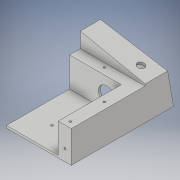
# Autodesk Inventor part: CPLRightOne
Saved by Autodesk Inventor 2019 (Build 230136000, 136)
## iProperties
Created: 2019-01-04
Part Number: CPLRightOne
Material: Generic
Document SubType Name: Modeling
Designer: james
Density: 1 g/cm^3
Appearance: Default
Author: james
Autodesk Inventor part; units mm, degrees
ref_plane "YZ Plane" through (0, 0, 0) normal (1, 0, 0) x (0, 1, 0)
ref_plane "XZ Plane" through (0, 0, 0) normal (0, 1, 0) x (-1, 0, 0)
ref_plane "XY Plane" through (0, 0, 0) normal (0, 0, 1) x (1, 0, 0)
sketch "Sketch1" plane through (0, 0, 0) normal (0, 1, 0) x (-1, 0, 0)
  line L0 (99.052281, 106.212918) -> (-21.597719, 106.212918)
  line L1 (-21.597719, 106.212918) -> (-21.597719, -39.837082)
  line L2 (-21.597719, -39.837082) -> (99.052281, -39.837082)
  line L3 (99.052281, -39.837082) -> (99.052281, 106.212918)
  point P0 (0, 0)
  dimension "d0" = 146.05
  dimension "d1" = 120.65
  constraints: 8 end point, 2 parallel, 1 horizontal, 1 perpendicular
  measures "d0" distance of L0.end L1.end
  measures "d1" distance of L1.end L2.end
extrude "Extrusion1" add sketch "Sketch1" along normal blind 5.08
sketch "Sketch2" plane through (21.597719, 0, 106.212918) normal (1, 0, 0) x (0, 0, -1)
  line L0 (0, 5.08) -> (146.05, 5.08) projected
  line L1 (146.05, 5.08) -> (140.97, 5.08)
  line L2 (140.97, 5.08) -> (140.97, 71.12)
  line L3 (140.97, 71.12) -> (146.05, 71.12)
  line L4 (146.05, 71.12) -> (146.05, 5.08)
  line L5 (0, 0) -> (146.05, 0) projected
  point P0 (106.212918, 0)
  dimension "d4" = 5.08
  dimension "d5" = 71.12
  constraints: 8 end point, 2 parallel, 1 horizontal, 1 perpendicular
  measures "d4" distance between parallel lines of L2 L4
  measures "d5" distance between parallel lines of L3 L5
extrude "Extrusion2" add sketch "Sketch2" against normal blind 120.65
sketch "Sketch3" plane through (-99.052281, 0, 106.212918) normal (0, 0, 1) x (1, 0, 0)
  line L0 (0, 5.08) -> (120.65, 5.08) projected
  line L1 (120.65, 5.08) -> (115.57, 5.08)
  line L2 (115.57, 5.08) -> (115.57, 71.12)
  line L3 (115.57, 71.12) -> (120.65, 71.12)
  line L4 (120.65, 71.12) -> (120.65, 5.08)
  line L5 (0, 0) -> (120.65, 0) projected
  point P0 (99.052281, 0)
  dimension "d8" = 5.08
  dimension "d9" = 71.12
  constraints: 8 end point, 2 parallel, 1 horizontal, 1 perpendicular
  measures "d8" distance between parallel lines of L4 L2
  measures "d9" distance between parallel lines of L3 L5
extrude "Extrusion3" add sketch "Sketch3" against normal blind 146.05
sketch "Sketch4" plane through (-99.052281, 0, 106.212918) normal (0, 0, 1) x (1, 0, 0)
  line L0 (115.57, 5.08) -> (115.57, 71.12) projected
  line L1 (115.57, 71.12) -> (120.65, 71.12) projected
  line L2 (115.57, 71.12) -> (139.7, 71.12)
  line L3 (139.7, 71.12) -> (139.7, 66.04)
  line L4 (139.7, 66.04) -> (115.57, 66.04)
  line L5 (115.57, 66.04) -> (115.57, 71.12)
  point P0 (99.052281, 0)
  dimension "d12" = 5.08
  dimension "d13" = 24.13
  constraints: 8 end point, 2 parallel, 1 horizontal, 1 perpendicular
  measures "d12" distance between parallel lines of L4 L2
  measures "d13" distance of L0.end L2.end
extrude "Extrusion4" add sketch "Sketch4" against normal blind 165.1
sketch "Sketch5" plane through (-99.052281, 0, -39.837082) normal (-1, 0, 0) x (0, 0, 1)
  line L0 (5.08, 5.08) -> (5.08, 71.12) projected
  line L1 (5.08, 71.12) -> (0, 71.12) projected
  line L2 (5.08, 71.12) -> (-19.05, 71.12)
  line L3 (-19.05, 71.12) -> (-19.05, 66.04)
  line L4 (-19.05, 66.04) -> (5.08, 66.04)
  line L5 (5.08, 66.04) -> (5.08, 71.12)
  point P0 (39.837082, 0)
  dimension "d16" = 5.08
  dimension "d17" = 24.13
  constraints: 8 end point, 2 parallel, 1 horizontal, 1 perpendicular
  measures "d16" distance between parallel lines of L4 L2
  measures "d17" distance of L0.end L2.end
extrude "Extrusion5" add sketch "Sketch5" against normal blind 139.7
sketch "Sketch7" plane through (-99.052281, 0, -58.887082) normal (0, 0, -1) x (-1, 0, 0)
  line L0 (-139.7, 71.12) -> (-144.78, 71.12)
  line L1 (-144.78, 71.12) -> (-144.78, 0)
  line L2 (-144.78, 0) -> (-139.7, 0)
  line L3 (-139.7, 0) -> (-139.7, 71.12)
  line L4 (-139.7, 71.12) -> (-139.7, 66.04) projected
  point P0 (-99.052281, 0)
  dimension "d26" = 5.08
  dimension "d27" = 0
  dimension "d28" = 71.12
  constraints: 8 end point, 2 parallel, 1 horizontal, 1 perpendicular
  measures "d26" distance between parallel lines of L1 L3
  measures "d27" distance between parallel lines of L4 L3
  measures "d28" distance between parallel lines of L0 L2
extrude "Extrusion7" add sketch "Sketch7" against normal blind 165.1
sketch "Sketch8" plane through (-99.052281, 0, -39.837082) normal (-1, 0, 0) x (0, 0, 1)
  line L0 (-77.47, 0) -> (-82.55, 0)
  line L1 (146.05, 0) -> (146.05, 5.08)
  line L2 (-77.47, 0) -> (-55.076473, 127)
  line L3 (-19.05, 0) -> (-19.05, 66.04)
  line L4 (-55.076473, 127) -> (-60.156473, 127)
  line L5 (-60.156473, 127) -> (-82.55, 0)
  point P0 (39.837082, 0)
  dimension "d31" = 5.08
  dimension "d32" = 228.6
  dimension "d33" = 10
  dimension "d34" = 5.08
  dimension "d35" = 127
  constraints: 8 end point, 2 horizontal
  measures "d31" distance of L0.start L0.end
  measures "d32" distance from line of L0.end L1
  measures "d33" angle of L2 L3
  measures "d34" distance of L2.end L4.end
  measures "d35" distance between parallel lines of L0 L4
extrude "Extrusion8" add sketch "Sketch8" against normal blind 144.78
sketch "Sketch9" plane through (-99.052281, 0, -39.837082) normal (-1, 0, 0) x (0, 0, 1)
  line L0 (-19.05, 0) -> (-19.05, 66.04) projected
  line L1 (-19.05, 66.04) -> (-24.13, 66.04)
  line L2 (-24.13, 66.04) -> (-24.13, 142.24)
  line L3 (-24.13, 142.24) -> (-19.05, 142.24)
  line L4 (-19.05, 142.24) -> (-19.05, 66.04)
  point P0 (39.837082, 0)
  dimension "d38" = 76.2
  dimension "d39" = 5.08
  constraints: 8 end point, 2 parallel, 1 horizontal, 1 perpendicular
  measures "d38" distance of L3.end L0.end
  measures "d39" distance between parallel lines of L2 L4
extrude "Extrusion9" add sketch "Sketch9" against normal blind 144.78
sketch "Sketch13" plane through (-99.052281, 71.12, -58.887082) normal (0, 0, 1) x (1, 0, 0)
  line L0 (0, 55.88) -> (0, -71.12)
  line L1 (0, -71.12) -> (120.65, -71.12)
  line L2 (0, 34.1884) -> (-78.886299, 34.1884)
  line L3 (0, 34.1884) -> (158.447464, 1.144718)
  line L4 (0, 34.1884) -> (0, 135.397645)
  line L5 (0, 135.397645) -> (157.416456, 135.397645)
  line L6 (157.416456, 135.397645) -> (158.447464, 1.144718)
  point P0 (99.052281, -71.12)
  dimension "d51" = 168.22
  constraints: 10 end point, 1 horizontal, 1 perpendicular, 1 point on line, 1 vertical
  measures "d51" angle of L2 L3
extrude "Extrusion13" cut sketch "Sketch13" against normal blind 114.6175
sketch "Sketch26" plane through (0, 5.08, 0) normal (0, 1, 0) x (1, 0, 0)
  line L0 (-99.052281, 34.757082) -> (-99.052281, -106.212918)
  line L1 (-99.052281, -106.212918) -> (16.517719, -106.212918)
  point P0 (0, 0)
  point P1 (-48.252281, -55.412918)
  dimension "d93" = 50.8
  dimension "d94" = 50.8
  measures "d93" distance from line of L0 point (-48.252, -55.413)
  measures "d94" distance from line of L1 point (-48.252, -55.413)
hole "Hole3" at (-48.252281, 5.08, 55.412918) direction (0, -1, 0) diameter 4.826 end through all
sketch "Sketch29" plane through (45.727719, 0, -58.887082) normal (1, 0, 0) x (0, 0, -1)
  line L0 (45.175195, 75.115022) -> (58.42, 0)
  line L1 (5.08, 73.952952) -> (45.175195, 73.952952)
  line L2 (5.08, 66.04) -> (5.08, 75.115022)
  line L3 (0, 66.04) -> (5.08, 66.04)
  line L4 (0, 66.04) -> (0, 0)
  line L5 (-19.05, 0) -> (58.42, 0)
  point P0 (-58.887082, 0)
  point P1 (36.026473, 127)
  point P2 (5.08, 142.24)
sketch "Sketch29 outline for Extrusion22" plane through (45.727719, 0, -58.887082) normal (1, 0, 0) x (0, 0, -1)
  line L0 (45.175195, 75.115022) -> (58.42, 0)
  line L1 (58.42, 0) -> (0, 0)
  line L2 (0, 0) -> (0, 66.04)
  line L3 (0, 66.04) -> (5.08, 66.04)
  line L4 (5.08, 66.04) -> (5.08, 75.115022)
  line L5 (5.08, 75.115022) -> (45.175195, 75.115022)
extrude "Extrusion22" add sketch "Sketch29 outline for Extrusion22" against normal blind 5.08
sketch "Sketch38" plane through (-99.052281, 105.3084, -98.73837) normal (0.2041544, 0.9789387, 0) x (0.9789387, -0.2041544, 0)
  line L0 (147.894856, -34.771288) -> (147.894856, 5.323907)
  line L1 (147.894856, 5.323907) -> (147.894856, -34.772919)
  line L2 (142.921848, -34.771288) -> (142.921848, 5.323907)
  line L3 (147.894856, -34.772919) -> (3.742348, -34.772919)
  line L4 (8.016815, -34.771288) -> (144.774553, -34.771288)
  line L5 (3.742348, -34.772919) -> (3.742348, -0.025087)
  line L6 (3.742348, -0.025087) -> (3.742348, 2.656747)
  line L7 (3.742348, 2.656747) -> (147.804186, 7.842673)
  line L8 (0, 5.08) -> (147.894856, 10.403907)
  line L9 (147.894856, 10.403907) -> (147.894856, 5.323907)
  line L10 (147.804186, 7.842673) -> (147.894856, 5.323907)
  point P0 (118.46528, -98.73837)
  constraints: 10 end point, 2 parallel, 2 vertical, 1 horizontal, 1 perpendicular, 4 other
extrude "Extrusion30" add sketch "Sketch38" against normal blind 5.08
sketch "Sketch40" plane through (-99.052281, 0, -39.837082) normal (-1, 0, 0) x (0, 0, 1)
  line L0 (0, 0) -> (0, 66.04)
  line L1 (-24.13, 66.04) -> (0, 66.04)
  line L2 (-24.13, 66.04) -> (-24.13, 105.3084)
  line L3 (-58.901288, 105.3084) -> (-77.47, 0)
  line L4 (-19.05, 105.3084) -> (-24.13, 105.3084)
  line L5 (-24.13, 104.544383) -> (-59.036005, 104.544383)
  line L6 (-24.13, 105.3084) -> (-59.036005, 104.544383)
  line L7 (146.05, 0) -> (0, 0)
  line L8 (-77.47, 0) -> (146.05, 0)
  line L9 (0, 0) -> (-77.47, 0)
  point P0 (39.837082, 0)
  constraints: 4 end point, 1 horizontal
extrude "Extrusion31" add sketch "Sketch40" against normal blind 5.08 contours L8 L3 L5 L2 L1 L0
sketch "Sketch41" plane through (-99.052281, 104.544383, -63.967082) normal (0, 0, -1) x (-1, 0, 0)
  line L0 (-3.66353, 0) -> (0, 0)
  line L1 (0, 0) -> (0, 0.764017)
  line L2 (0, 0.764017) -> (-3.66353, 0)
  point P0 (-99.052281, -104.544383)
  point P1 (-5.08, -5.484693)
extrude "Extrusion32" add sketch "Sketch41" along normal blind 36.83
sketch "Sketch43" plane through (-99.052281, 71.12, -58.887082) normal (0, 0, 1) x (1, 0, 0)
  line L0 (5.08, 33.128983) -> (3.66353, 33.424383)
  line L1 (5.08, 33.424383) -> (5.08, 33.128983)
  line L2 (3.66353, 33.424383) -> (5.08, 33.424383)
  point P0 (99.052281, -71.12)
extrude "Extrusion33" cut sketch "Sketch43" against normal blind 41.5925
sketch "Sketch44" plane through (40.647719, 0, 106.212918) normal (-1, 0, 0) x (0, 0, 1)
  line L0 (0, 66.04) -> (-170.18, 66.04)
  line L1 (-170.18, 66.04) -> (-142.520317, 66.04)
  line L2 (-142.520317, 66.04) -> (-142.520317, 48.69089)
  line L3 (-142.520317, 48.69089) -> (-170.18, 66.04)
  point P0 (-106.212918, 0)
  constraints: 6 end point, 1 point on line, 1 vertical
extrude "Extrusion34" add sketch "Sketch44" along normal blind 135.255
sketch "Sketch47" plane through (-99.052281, 0, 106.212918) normal (0, 0, 1) x (1, 0, 0)
  line L0 (139.7, 66.04) -> (120.65, 66.04)
  line L1 (139.741198, 66.04) -> (120.65, 66.04)
  line L2 (120.65, 66.04) -> (139.741198, 59.182182)
  line L3 (139.741198, 59.182182) -> (139.741198, 66.04)
  line L4 (139.7, 0) -> (139.7, 70.985145)
  point P0 (99.052281, 0)
  constraints: 6 end point, 1 collinear, 1 parallel
extrude "Extrusion35" add sketch "Sketch47" against normal blind 143.1925
sketch "Sketch19" plane through (-99.052281, 71.12, -34.757082) normal (0, 1, 0) x (1, 0, 0)
  line L0 (144.78, 24.13) -> (0, 24.13) projected
  line L1 (115.57, -140.97) -> (115.57, 0) projected
  point P0 (99.052281, -34.757082)
  point P1 (130.175, -52.07)
  point P2 (130.175, -128.27)
  dimension "d63" = 76.2
  dimension "d64" = 14.605
  dimension "d65" = 14.605
  dimension "d66" = 76.2
  measures "d63" distance of point (130.175, -128.27) point (130.175, -52.07)
  measures "d64" distance from line of L1 point (130.175, -128.27)
  measures "d65" distance from line of L1 point (130.175, -52.07)
  measures "d66" distance from line of point (130.175, -52.07) L0
hole "Hole1" at (31.122719, 71.12, 17.312918) at (31.122719, 71.12, 93.512918) direction (0, -1, 0) diameter 4.826 end through all
sketch "Sketch20" plane through (-99.052281, 71.12, -34.757082) normal (0, 1, 0) x (1, 0, 0)
  line L0 (115.57, 0) -> (0, 0) projected
  circle A0 centre (130.175, -52.07) radius 2.413 projected
  point P0 (99.052281, -34.757082)
  point P1 (63.5, 14.605)
  dimension "d74" = 14.605
  dimension "d75" = 66.675
  measures "d74" distance from line of point (63.5, 14.605) L0
  measures "d75" horizontal distance of A0.centre point (63.5, 14.605)
hole "Hole2" at (-35.552281, 71.12, -49.362082) direction (0, -1, 0) diameter 4.826 end through all
sketch "Sketch48" plane through (-99.052281, 0, 106.212918) normal (0, 0, 1) x (1, 0, 0)
  line L0 (5.08, 66.04) -> (139.7, 66.04)
  line L1 (120.65, 66.04) -> (139.7, 59.196981)
  line L2 (139.7, 59.196981) -> (139.7, 0)
  line L3 (120.65, 0) -> (120.65, 66.04)
  line L4 (139.7, 0) -> (120.65, 0)
  line L5 (0, 0) -> (144.78, 0)
  point P0 (99.052281, 0)
  constraints: 2 end point, 1 collinear
extrude "Extrusion36" add sketch "Sketch48" against normal blind 5.08
sketch "Sketch49" plane through (-99.052281, 5.08, -34.757082) normal (-1, 0, 0) x (0, 0, 1)
  line L0 (0, 0) -> (0, 66.04) projected
  line L1 (140.97, -5.08) -> (-87.63, -5.08) projected
  point P0 (34.757082, -5.08)
  point P1 (-50.8, 20.32)
  point P2 (-50.8, 45.72)
  dimension "d152" = 50.8
  dimension "d153" = 50.8
  dimension "d154" = 25.4
  dimension "d155" = 25.4
  measures "d152" distance from line of L0 point (-50.8, 45.72)
  measures "d153" distance from line of L0 point (-50.8, 20.32)
  measures "d154" distance from line of L1 point (-50.8, 20.32)
  measures "d155" distance of point (-50.8, 45.72) point (-50.8, 20.32)
hole "Hole6" at (-99.052281, 25.4, -85.557082) at (-99.052281, 50.8, -85.557082) direction (1, 0, 0) diameter 4.826 depth 25.4 tip angle 118
sketch "Sketch50" plane through (-99.052281, 0, 106.212918) normal (0, 0, 1) x (1, 0, 0)
  line L0 (0, 0) -> (144.78, 0) projected
  line L1 (115.57, 5.08) -> (115.57, 71.12) projected
  point P0 (99.052281, 0)
  point P1 (130.81, 25.4)
  dimension "d163" = 25.4
  dimension "d164" = 15.24
  measures "d163" distance from line of point (130.81, 25.4) L0
  measures "d164" distance from line of L1 point (130.81, 25.4)
hole "Hole7" at (31.757719, 25.4, 106.212918) direction (0, 0, -1) diameter 4.826 depth 25.4 tip angle 118
sketch "Sketch51" plane through (45.727719, 75.115022, -58.887082) normal (0.2041544, 0.9789387, 0) x (0.9789387, -0.2041544, 0)
  line L0 (-147.894856, 44.931288) -> (0, 50.255195)
  line L1 (0, 0) -> (-147.894856, 0)
  line L2 (0, 50.255195) -> (0, 0)
  point P0 (-29.429576, -58.887082)
  point P1 (-34.205528, 24.13)
  dimension "d172" = 24.87775
  dimension "d173" = 24.13
  dimension "d174" = 34.20553
  measures "d172" distance from line of L0 point (-34.206, 24.13)
  measures "d173" distance from line of L1 point (-34.206, 24.13)
  measures "d174" distance from line of L2 point (-34.206, 24.13)
hole "Hole8" at (12.242604, 82.098229, -83.017082) direction (-0.2041544, -0.9789387, 0) diameter 15.875 depth 25.4 tip angle 118.1875
sketch "Sketch52" plane through (-99.052281, 5.08, -34.757082) normal (0, 0, 1) x (1, 0, 0)
  circle A0 centre (83.137068, 28.704927) radius 19.05
  point P0 (99.052281, -5.08)
  dimension "d182" = 38.1
  constraints: 1 centre point
  measures "d182" diameter of A0
extrude "Extrusion37" cut sketch "Sketch52" against normal blind 25.4
equation "\"d0\" = CPDLengthHole"
equation "\"d1\" = CPDWidthHole"
equation "\"d2\" = WallWidth"
equation "\"d4\" = WallWidth"
equation "\"d5\" = CPDeckHeight"
equation "\"d6\" = CPDWidthHole"
equation "\"d8\" = WallWidth"
equation "\"d9\" = CPDeckHeight"
equation "\"d10\" = CPDLengthHole"
equation "\"d12\" = WallWidth"
equation "\"d13\" = WallWidth + ControlPlateShelfLength"
equation "\"d14\" = CPDLengthHole + ControlPlateShelfLength"
equation "\"d16\" = WallWidth"
equation "\"d17\" = WallWidth + ControlPlateShelfLength"
equation "\"d18\" = CPDWidthHole + ControlPlateShelfLength"
equation "\"d26\" = WallWidth"
equation "\"d28\" = CPDeckHeight"
equation "\"d31\" = WallWidth"
equation "\"d32\" = PartLength"
equation "\"d33\" = EdgeAngle"
equation "\"d34\" = WallWidth"
equation "\"d35\" = DSBackHeight"
equation "\"d39\" = WallWidth"
equation "\"d51\" = MainAngle"
equation "\"d122\" = WallWidth"
equation "\"d138\" = WallWidth"
equation "\"d140\" = WallWidth"
equation "\"d64\" = ControlHoleBoltHoleMid + WallWidth"
equation "\"d65\" = ControlHoleBoltHoleMid + WallWidth"
equation "\"d74\" = ControlHoleBoltHoleMid + WallWidth"
equation "\"d150\" = WallWidth"
equation "\"DSLength\" = 1371.6"
equation "\"DSWidth\" = 304.8"
equation "\"DCDeckHeight\" = 76.2"
equation "\"WallWidth\" = 5.08"
equation "\"EdgeAngle\" = 10deg"
equation "\"LengthCuts\" = 152.4"
equation "\"WidthCuts\" = 50.8"
equation "\"PartLength\" = 228.6"
equation "\"PartWidth\" = 152.4"
equation "\"BoltHoldDiam\" = 6.35"
equation "\"ControlPlateLength\" = 228.6"
equation "\"ControlPlateWidth\" = 228.6"
equation "\"ControlPlateShelfLength\" = 19.05"
equation "\"ControlHoleLength\" = 190.5"
equation "\"ControlHoleWidth\" = 190.5"
equation "\"ControlHoleFromSide\" = 63.5"
equation "\"ControlHoleBoltHoleMid\" = 9.525"
equation "\"CPDeckHeight\" = 71.12"
equation "\"CPFromSide\" = 63.5"
equation "\"CPFromBack\" = 63.5"
equation "\"DU1CHWidth\" = 69.85"
equation "\"DU1CHLength\" = 146.05"
equation "\"ControlPlateScrewLength\" = 76.2"
equation "\"DSBackHeight\" = 127"
equation "\"BackShelf\" = 25.4"
equation "\"MainAngle\" = 168.22deg"
equation "\"CPDWidthHole\" = 120.65"
equation "\"CPDLengthHole\" = 146.05"
equation "\"DownBackHeight\" = 130.7084"
body "Solid1"
